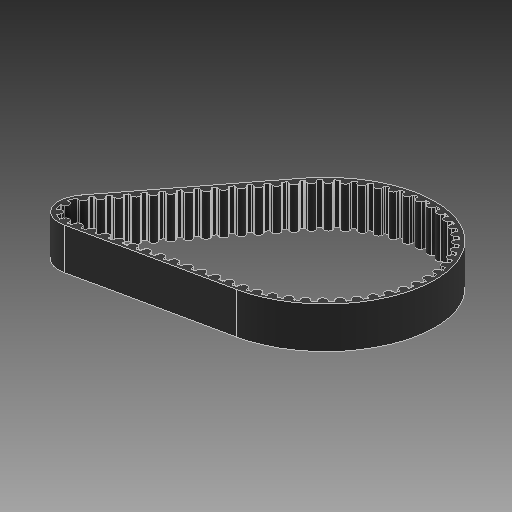
# Autodesk Inventor part: Belt Generator
Saved by Autodesk Inventor 2023 (Build 270158000, 158)
## iProperties
RuleStatus: InUse
Created: 2020-06-05
Material: Rubber
Document SubType Name: Modeling
Density: 0.93 g/cm^3
Appearance: Rubber - Black
AfterAnyiPropertyChange0: GT2toHTD
AfterAnyParamChange0: GT2toHTD
PartBodyChanged0: GT2toHTD
Autodesk Inventor part; units mm, degrees
ref_plane "YZ Plane" through (0, 0, 0) normal (1, 0, 0) x (0, 1, 0)
ref_plane "XY Plane" through (0, 0, 0) normal (0, 0, 1) x (1, 0, 0)
sketch "top teeth placement" plane through (0, 0, 0) normal (0, 1, 0) x (-1, 0, 0)
  arc A0 (3.9614, -8.6889) -> (3.9614, 8.6889) centre (0, 0) ccw construction
  line L0 (3.9614, -8.6889) -> (-53.2122, -34.7554) construction
  line L1 (3.9614, 8.6889) -> (-53.2122, 34.7554) construction
  arc A1 (-53.2122, 34.7554) -> (-53.2122, -34.7554) centre (-69.0579, 0) ccw construction
  arc A2 (3.9614, -8.6889) -> (7.7751, -5.5441) centre (0, 0) ccw construction
  arc A3 (-59.971, -37.1006) -> (-53.2122, -34.7554) centre (-69.0579, 0) ccw construction
  arc A4 (-64.8913, -37.9693) -> (-59.971, -37.1006) centre (-69.0579, 0) ccw construction
  line L2 (3.9614, -8.6889) -> (0, 0) construction
  line L3 (0, 0) -> (7.7751, -5.5441) construction
  line L4 (-59.971, -37.1006) -> (-69.0579, 0) construction
  line L5 (-69.0579, 0) -> (-64.8913, -37.9693) construction
  point P0 (-0.5881, -10.7631)
  point P1 (-5.1375, -12.8372)
  point P2 (-9.687, -14.9114)
  point P3 (-14.2365, -16.9856)
  point P4 (-18.786, -19.0598)
  point P5 (-23.3354, -21.134)
  point P6 (1.0773, 10.0038)
  point P7 (-3.4722, 12.078)
  point P8 (-27.8849, -23.2082)
  point P9 (-32.4344, -25.2824)
  point P10 (-36.9839, -27.3566)
  point P11 (-41.5333, -29.4308)
  point P12 (-46.0828, -31.505)
  point P13 (-50.6323, -33.5792)
  point P14 (-55.1817, -35.6534)
  dimension "pitch" = 5
  dimension "r_d35" = 65
  dimension "r_d36" = 20
  dimension "d17" = 19.0986
  dimension "d18" = 76.3944
  dimension "d30" = 5
  dimension "d35" = 62.8354
  dimension "d36" = 21.8303
  dimension "d39" = 30
  dimension "d41" = 5
  dimension "d44" = 7.1646
  dimension "d45" = 152.6789
  dimension "d48" = 7.5
  dimension "d50" = 5
  dimension "d52" = 3.1697
  dimension "d62" = 5
  dimension "d71" = 69.0579
  constraints: 12 end point, 11 point on circle, 5 centre point, 4 coincident, 4 tangent, 3 concentric, 1 horizontal alignment, 1 point on line, 20 other
  measures "d17" diameter of A0
  measures "d18" diameter of A1
  measures "d30" distance of L2.start point (-0.588, -10.763)
  measures "d35" distance of L0.start L0.end
  measures "d52" distance of point (1.077, 10.004) L1.start
  measures "d62" distance of point (1.077, 10.004) point (-3.472, 12.078)
  measures "d71" distance of A1.centre point (0, 0)
sketch "Tooth Profile" plane through (0, 0, 0) normal (0, 1, 0) x (-1, 0, 0)
  line L0 (-59.971, -37.1006) -> (-69.0579, 0) construction
  arc A0 (-53.2122, 34.7554) -> (-53.2122, -34.7554) centre (-69.0579, 0) ccw construction
  line L1 (3.9614, -8.6889) -> (-53.2122, -34.7554) construction
  line L2 (3.9614, 8.6889) -> (-53.2122, 34.7554) construction
  arc A1 (4.2626, -6.2621) -> (1.9319, -7.3247) centre (3.4049, -7.4682) ccw
  arc A2 (4.9754, -7.1877) -> (5.4482, -7.3829) centre (5.303, -7.0644) ccw
  line L3 (5.4482, -7.3829) -> (2.0005, -8.9548)
  line L4 (3.1036, -7.892) -> (3.513, -7.7053) construction
  arc A3 (4.9754, -7.1877) -> (4.2626, -6.2621) centre (3.1036, -7.892) ccw
  arc A4 (2.0005, -8.9548) -> (2.1632, -8.4699) centre (1.8553, -8.6363) ccw
  arc A5 (1.9319, -7.3247) -> (2.1632, -8.4699) centre (3.9225, -7.5187) ccw
  line L5 (5.8631, -8.2928) -> (2.4153, -9.8647)
  line L6 (5.8631, -8.2928) -> (5.4482, -7.3829)
  line L7 (2.4153, -9.8647) -> (2.0005, -8.9548)
  line L8 (2.791, -6.1216) -> (3.7243, -8.1689) construction
  line L9 (3.513, -7.7053) -> (3.9225, -7.5187) construction
  arc A6 (-0.9522, 8.6397) -> (1.3785, 7.577) centre (0.5208, 8.7832) ccw
  arc A7 (-0.721, 9.7848) -> (-0.8837, 10.2697) centre (-1.0288, 9.9513) ccw
  line L10 (-0.8837, 10.2697) -> (2.5641, 8.6978)
  line L11 (1.0383, 8.8336) -> (0.6289, 9.0203) construction
  arc A8 (-0.721, 9.7848) -> (-0.9522, 8.6397) centre (1.0383, 8.8336) ccw
  arc A9 (2.5641, 8.6978) -> (2.0913, 8.5026) centre (2.4189, 8.3794) ccw
  arc A10 (1.3785, 7.577) -> (2.0913, 8.5026) centre (0.2194, 9.2069) ccw
  line L12 (-0.4688, 11.1796) -> (2.9789, 9.6077)
  line L13 (-0.4688, 11.1796) -> (-0.8837, 10.2697)
  line L14 (2.9789, 9.6077) -> (2.5641, 8.6978)
  line L15 (-0.0932, 7.4365) -> (0.8402, 9.4838) construction
  line L16 (0.6289, 9.0203) -> (0.2194, 9.2069) construction
  arc A11 (-59.2226, -34.7726) -> (-61.7106, -35.3819) centre (-60.2901, -35.7976) ccw
  arc A12 (-58.6948, -35.8148) -> (-58.2668, -36.0948) centre (-58.35, -35.7548) ccw
  line L17 (-58.2668, -36.0948) -> (-61.9471, -36.9962)
  line L18 (-60.6652, -36.1577) -> (-60.2281, -36.0507) construction
  arc A13 (-58.6948, -35.8148) -> (-59.2226, -34.7726) centre (-60.6652, -36.1577) ccw
  arc A14 (-61.9471, -36.9962) -> (-61.6969, -36.5501) centre (-62.0304, -36.6563) ccw
  arc A15 (-61.7106, -35.3819) -> (-61.6969, -36.5501) centre (-59.7911, -35.9436) ccw
  line L19 (-58.0289, -37.0661) -> (-61.7092, -37.9675)
  line L20 (-58.0289, -37.0661) -> (-58.2668, -36.0948)
  line L21 (-61.7092, -37.9675) -> (-61.9471, -36.9962)
  line L22 (-60.6422, -34.3601) -> (-60.1069, -36.5455) construction
  line L23 (-60.2281, -36.0507) -> (-59.7911, -35.9436) construction
  line L24 (-59.7375, -37.0434) -> (-60.2045, -37.1578) construction
  dimension "d170" = 1.48
  dimension "d172" = 0.35
  dimension "d173" = 0.5715
  dimension "d175" = 0.45
  dimension "d176" = 2
  dimension "d177" = 1
  dimension "d178" = 2.25
  dimension "d185" = 1.48
  dimension "d186" = 0.35
  dimension "d187" = 0.45
  dimension "d188" = 2
  dimension "d189" = 1
  dimension "d190" = 2.25
  dimension "d192" = 0.5715
  dimension "d193" = 3.1697
  dimension "d194" = 1.48
  dimension "d195" = 0.35
  dimension "d196" = 0.45
  dimension "d197" = 2
  dimension "d198" = 1
  dimension "d199" = 2.25
  dimension "d200" = 0.5715
  dimension "d206" = 3.25
  dimension "d207" = 3.0908
  constraints: 44 end point, 33 point on circle, 19 tangent, 15 centre point, 13 perpendicular, 8 point on line, 5 parallel, 4 midpoint, 3 collinear, 3 equal radius, 2 coincident
  measures "d170" radius of A1
  measures "d172" radius of A2
  measures "d173" distance between parallel lines of L1 L3
  measures "d175" distance of L4.start L4.end
  measures "d176" radius of A3
  measures "d177" distance between parallel lines of L5 L3
  measures "d178" distance of L8.start L8.end
  measures "d185" radius of A6
  measures "d186" radius of A7
  measures "d187" distance of L11.start L16.start
  measures "d188" radius of A8
  measures "d189" distance between parallel lines of L12 L10
  measures "d190" distance of L15.start L15.end
  measures "d192" distance between parallel lines of L2 L10
  measures "d193" distance from line of L2.start L15
  measures "d194" radius of A11
  measures "d195" radius of A12
  measures "d196" distance of L18.start L23.start
  measures "d197" radius of A13
  measures "d198" distance between parallel lines of L19 L17
  measures "d199" distance of L22.start L22.end
  measures "d200" distance between parallel lines of L24 L17
  measures "d207" distance of A4.end A2.start
extrude "Top/Left Base Tooth" add sketch "Tooth Profile" against normal mid plane 15 contours A3 A2 L3 A4 A5 A1 | L6 L5 L7 L3
pattern_sketch "Top Teeth" of "Top/Left Base Tooth" from (-3.9614, 0, -8.6889) copies at (0.5881, 0, -10.7631) at (5.1375, 0, -12.8372) at (9.687, 0, -14.9114) at (14.2365, 0, -16.9856) at (18.786, 0, -19.0598) at (23.3354, 0, -21.134) at (27.8849, 0, -23.2082) at (32.4344, 0, -25.2824) at (36.9839, 0, -27.3566) at (41.5333, 0, -29.4308) at (46.0828, 0, -31.505) at (50.6323, 0, -33.5792) at (55.1817, 0, -35.6534)
pattern_circular "Left Teeth" count 4 over 120 about axis through (0, 0, 0) along (0, 1, 0) of "Top/Left Base Tooth"
extrude "Right Base Tooth" add sketch "Tooth Profile" along normal mid plane 15 contours A13 A12 L17 A14 A15 A11 | L20 L19 L21 L17
pattern_circular "Right Teeth" count 30 over 217.5 about axis through (69.0579, 0, 0) along (0, -1, 0) of "Right Base Tooth"
sketch "bottom teeth placement" plane through (0, 0, 0) normal (0, 1, 0) x (-1, 0, 0)
  arc A0 (3.9614, -8.6889) -> (3.9614, 8.6889) centre (0, 0) ccw construction
  line L0 (3.9614, -8.6889) -> (-53.2122, -34.7554) construction
  line L1 (3.9614, 8.6889) -> (-53.2122, 34.7554) construction
  arc A1 (-53.2122, 34.7554) -> (-53.2122, -34.7554) centre (-69.0579, 0) ccw construction
  point P0 (0.1674, 10.4186)
  point P1 (-4.3821, 12.4928)
  point P2 (-8.9315, 14.567)
  point P3 (-13.481, 16.6412)
  point P4 (-18.0305, 18.7154)
  point P5 (-22.58, 20.7896)
  point P6 (-27.1294, 22.8638)
  point P7 (-31.6789, 24.938)
  point P8 (-36.2284, 27.0122)
  point P9 (-40.7779, 29.0864)
  point P10 (-45.3273, 31.1606)
  point P11 (-49.8768, 33.2348)
  point P12 (-54.4263, 35.309)
  dimension "d144" = 3
  dimension "d147" = 21
  dimension "pitch" = 5
  dimension "d123" = 19.0986
  dimension "d124" = 76.3944
  dimension "d126" = 62.8354
  dimension "d127" = 21.8303
  dimension "d131" = 152.6789
  dimension "d134" = 4.1697
  dimension "d135" = 5
  dimension "d136" = 69.0579
  constraints: 4 end point, 4 point on circle, 4 tangent, 2 centre point, 2 coincident, 1 horizontal alignment, 1 point on line, 13 other
  measures "d123" diameter of A0
  measures "d124" diameter of A1
  measures "d126" distance of L0.start L0.end
  measures "d134" distance of point (0.167, 10.419) L1.start
  measures "d135" distance of point (0.167, 10.419) point (-4.382, 12.493)
  measures "d136" distance of A1.centre point (0, 0)
extrude "Bottom Base Tooth" add sketch "Tooth Profile" along normal mid plane 15 contours A8 A7 L10 A9 A10 A6 | L13 L12 L14 L10
pattern_sketch "Bottom Teeth" of "Bottom Base Tooth" from (-0.1674, 0, 10.4186) copies at (4.3821, 0, 12.4928) at (8.9315, 0, 14.567) at (13.481, 0, 16.6412) at (18.0305, 0, 18.7154) at (22.58, 0, 20.7896) at (27.1294, 0, 22.8638) at (31.6789, 0, 24.938) at (36.2284, 0, 27.0122) at (40.7779, 0, 29.0864) at (45.3273, 0, 31.1606) at (49.8768, 0, 33.2348) at (54.4263, 0, 35.309)
sketch "Sketch8" plane through (0, 0, 0) normal (0, 1, 0) x (-1, 0, 0)
  arc A0 (3.9614, -8.6889) -> (3.9614, 8.6889) centre (0, 0) ccw construction
  line L0 (3.9614, -8.6889) -> (-53.2122, -34.7554) construction
  line L1 (3.9614, 8.6889) -> (-53.2122, 34.7554) construction
  arc A1 (-53.2122, 34.7554) -> (-53.2122, -34.7554) centre (-69.0579, 0) ccw construction
  arc A2 (4.3632, -9.5701) -> (4.3632, 9.5701) centre (0, 0) ccw
  line L2 (4.3632, -9.5701) -> (-52.8104, -35.6367)
  arc A3 (-52.8104, 35.6367) -> (-52.8104, -35.6367) centre (-69.0579, 0) ccw
  line L3 (-52.8104, 35.6367) -> (4.3632, 9.5701)
  arc A4 (3.7243, -8.1689) -> (3.7243, 8.1689) centre (0, 0) ccw
  line L4 (3.7243, -8.1689) -> (-53.4493, -34.2354)
  arc A5 (-53.4493, 34.2354) -> (-53.4493, -34.2354) centre (-69.0579, 0) ccw
  line L5 (-53.4493, 34.2354) -> (3.7243, 8.1689)
  dimension "d201" = 0.5715
  dimension "d202" = 1.54
  constraints: 8 end point, 8 point on circle, 4 centre point, 6 other
  measures "d201" radial gap between concentric circles of A0 A4
  measures "d202" distance between parallel lines of L2 L4
extrude "Extrusion7" add sketch "Sketch8" along normal mid plane 15
equation "\"pitch\" = 5"
equation "\"r_d36\" = 20"
equation "\"d30\" = pitch"
equation "\"d41\" = pitch"
equation "\"d44\" = pitch + r_d35 - d35"
equation "\"d50\" = pitch"
equation "\"d62\" = pitch"
equation "\"d144\" = 3"
equation "\"d147\" = 21"
equation "\"pulley_1_angle\" = 30deg"
equation "\"pulley_2_angle\" = 7.5deg"
equation "\"d108\" = 5"
equation "\"d156\" = 5"
equation "\"center_distance\" = 69.05787"
equation "\"gt2_pld\" = 0.5715"
equation "\"missing_tooth_bottom_right_round\" = 0"
equation "\"missing_tooth_bottom_right_straight\" = 0"
equation "\"missing_tooth_bottom_left\" = 0"
equation "\"belt_width\" = 15"
equation "\"ThreeMM\" = 3"
body "Solid3"
